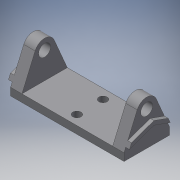
# Autodesk Inventor part: EpoxyFiberMountBase
Saved by Autodesk Inventor 2019 (Build 230136000, 136)
## iProperties
Created: 2019-05-24
Part Number: EpoxyFiberMountBase
Material: Generic
Document SubType Name: Modeling
Designer: aorfi
Density: 1 g/cm^3
Appearance: Default
Author: aorfi
Autodesk Inventor part; units mm, degrees
ref_plane "YZ Plane" through (0, 0, 0) normal (1, 0, 0) x (0, 1, 0)
ref_plane "XZ Plane" through (0, 0, 0) normal (0, 1, 0) x (-1, 0, 0)
ref_plane "XY Plane" through (0, 0, 0) normal (0, 0, 1) x (1, 0, 0)
sketch "Sketch1" plane through (0, 0, 0) normal (0, 1, 0) x (-1, 0, 0)
  line L0 (-15, 6) -> (15, 6)
  line L1 (15, 6) -> (15, -6)
  line L2 (15, -6) -> (-15, -6)
  line L3 (-15, -6) -> (-15, 6)
  line L4 (-15, 6) -> (15, -6) construction
  line L5 (15, 6) -> (-15, -6) construction
  point P0 (0, 0)
  dimension "d0" = 12
  dimension "d1" = 30
  constraints: 12 end point, 2 midpoint, 2 parallel, 1 horizontal, 1 perpendicular
  measures "d0" distance of L0.end L1.end
  measures "d1" distance of L0.start L0.end
extrude "Extrusion1" add sketch "Sketch1" along normal mid plane 2
sketch "Sketch2" plane through (-15, -1, 6) normal (-1, 0, 0) x (0, 0, 1)
  circle A0 centre (-6, 9) radius 1.5875
  circle A1 centre (-6, 9) radius 2.75
  line L0 (-8.5267, 10.0854) -> (-12, 2)
  line L1 (0, 0) -> (0, 2) projected
  line L2 (-12, 2) -> (0, 2)
  line L3 (0, 2) -> (-3.4733, 10.0854)
  point P0 (-6, 1)
  dimension "d4" = 3.175
  dimension "d5" = 5.5
  dimension "d6" = 7
  constraints: 6 end point, 2 centre point, 2 point on circle, 2 tangent, 1 coincident, 1 perpendicular, 1 vertical alignment
  measures "d4" diameter of A0
  measures "d5" diameter of A1
  measures "d6" distance from line of L2 A0.centre
extrude "Extrusion2" add sketch "Sketch2" against normal blind 3
mirror "Mirror1" about plane through (0, 0, 0) normal (1, 0, 0) of "Extrusion2"
sketch "Sketch3" plane through (0, 1, 0) normal (0, 1, 0) x (1, 0, 0)
  circle A0 centre (0, -3.4544) radius 1.0922 projected
  circle A1 centre (0, 3.4544) radius 1.0922 projected
  point P0 (-3.455, 0)
  point P1 (3.455, 0)
extrude "Extrusion4" cut sketch "Sketch3" against normal through all
sketch "Sketch5" plane through (15, -1, 6) normal (1, 0, 0) x (0, 0, -1)
  line L0 (8.5267, 10.0854) -> (12, 2) projected
  line L1 (12, 2) -> (8.5267, 10.0854) projected
  line L2 (0.9727, 4.2642) -> (0.4323, 3.0064)
  line L3 (0, 2) -> (3.4733, 10.0854) projected
  circle A0 centre (6, 9) radius 1.5875 projected
  circle A1 centre (6, 9) radius 2.75 construction
  line L4 (6.7482, 5.2835) -> (10.0744, 6.4827)
  line L5 (0.4323, 3.0064) -> (10.0744, 6.4827)
  arc A2 (8.5267, 10.0854) -> (3.4733, 10.0854) centre (6, 9) ccw projected
  line L6 (9.679, 7.4031) -> (10.0744, 6.4827)
  line L7 (0.9727, 4.2642) -> (9.679, 7.4031)
  line L8 (12, 0) -> (0, 0) projected
  point P0 (6, 1)
  dimension "d23" = 1
  dimension "d24" = 3.0064
  constraints: 11 end point, 2 collinear, 2 point on line, 1 centre point, 1 coincident, 1 concentric, 1 parallel, 1 tangent
  measures "d23" distance between parallel lines of L4 L7
  measures "d24" distance from line of L8 L2.end
extrude "Extrusion5" add sketch "Sketch5" along normal blind 1 contours L0 L4 L5 L2 L7
mirror "Mirror2" about plane through (0, 0, 0) normal (1, 0, 0) of "Extrusion5"
body "Solid1"
